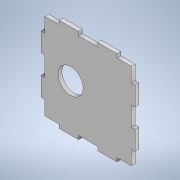
# Autodesk Inventor part: Top
Saved by Autodesk Inventor 2020 (Build 240168000, 168)
## iProperties
Created: 2020-12-28
Part Number: Top
Material: Generic
Document SubType Name: Modeling
Designer: solar
Density: 1 g/cm^3
Appearance: Default
Author: solar
Autodesk Inventor part; units mm, degrees
ref_plane "YZ Plane" through (0, 0, 0) normal (1, 0, 0) x (0, 1, 0)
ref_plane "XZ Plane" through (0, 0, 0) normal (0, 1, 0) x (-1, 0, 0)
ref_plane "XY Plane" through (0, 0, 0) normal (0, 0, 1) x (1, 0, 0)
sketch "Sketch1" plane through (0, 0, 0) normal (0, 0, 1) x (1, 0, 0)
  line L0 (-75, -15.375) -> (-69, -15.375)
  line L1 (-69, -46.125) -> (-75, -46.125)
  line L2 (-69, 46.125) -> (-75, 46.125)
  line L3 (-75, 15.375) -> (-69, 15.375)
  line L4 (-69, 46.125) -> (-69, 69)
  line L5 (-75, 46.125) -> (-75, 15.375)
  line L6 (-69, 15.375) -> (-69, -15.375)
  line L7 (-75, -15.375) -> (-75, -46.125)
  line L8 (-69, -46.125) -> (-69, -69)
  line L9 (0, 0) -> (0, 15.375)
  line L10 (0, 0) -> (0, -46.125)
  line L11 (69, 15.375) -> (69, -15.375)
  line L12 (75, 15.375) -> (69, 15.375)
  line L13 (75, 46.125) -> (75, 15.375)
  line L14 (69, 46.125) -> (75, 46.125)
  line L15 (69, 46.125) -> (69, 69)
  line L16 (75, -15.375) -> (69, -15.375)
  line L17 (75, -15.375) -> (75, -46.125)
  line L18 (69, -46.125) -> (75, -46.125)
  line L19 (69, -46.125) -> (69, -69)
  line L20 (0, 0) -> (92.4518, 92.4518)
  line L21 (0, 0) -> (102.0745, -102.0745)
  line L22 (-15.375, 75) -> (-15.375, 69)
  line L23 (-46.125, 69) -> (-46.125, 75)
  line L24 (-15.375, 75) -> (-46.125, 75)
  line L25 (-46.125, 69) -> (-69, 69)
  line L26 (15.375, 69) -> (-15.375, 69)
  line L27 (15.375, 75) -> (15.375, 69)
  line L28 (46.125, 75) -> (15.375, 75)
  line L29 (46.125, 69) -> (46.125, 75)
  line L30 (46.125, 69) -> (69, 69)
  line L31 (46.125, -69) -> (46.125, -75)
  line L32 (46.125, -75) -> (15.375, -75)
  line L33 (46.125, -69) -> (69, -69)
  line L34 (-15.375, -75) -> (-15.375, -69)
  line L35 (15.375, -75) -> (15.375, -69)
  line L36 (15.375, -69) -> (-15.375, -69)
  line L37 (-15.375, -75) -> (-46.125, -75)
  line L38 (-46.125, -69) -> (-46.125, -75)
  line L39 (-46.125, -69) -> (-69, -69)
  line L40 (0, 0) -> (-28, 0)
  circle A0 centre (-28, 0) radius 20
  point P0 (0, 0)
  point P1 (0, 0)
  point P2 (-69, -75)
  point P3 (-69, 75)
  point P4 (69, -75)
  point P5 (69, 75)
  dimension "d1" = 28
  dimension "d2" = 40
  constraints: 82 end point, 18 symmetric about line, 3 point on line, 2 vertical, 1 centre point, 1 coincident, 1 perpendicular
  measures "d1" distance of L9.start L40.end
  measures "d2" diameter of A0
extrude "Extrusion1" add sketch "Sketch1" along normal blind 6
body "Solid1"
